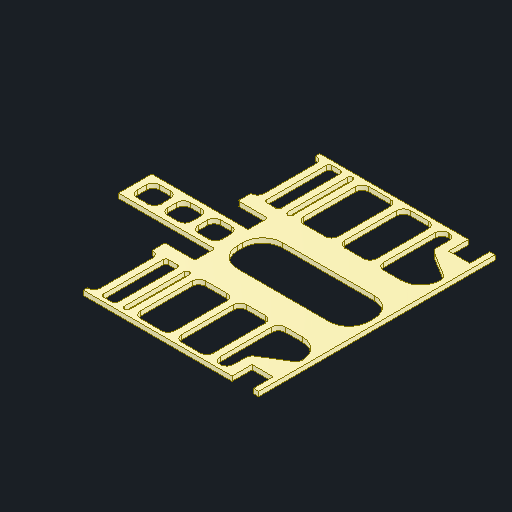
# Autodesk Inventor part: base
Saved by Autodesk Inventor 2023 (Build 270158000, 158)
## iProperties
Created: 2024-04-29
Part Number: base
Material: Nylon 6/6
Document SubType Name: Modeling
Designer: szymo
Density: 1.13 g/cm^3
Appearance: Nylon 6
Mass: 42.7646 g
Surface Area: 306.54 cm^2
Volume: 37.8447 cm^3
Author: szymo
Autodesk Inventor part; units mm, degrees
ref_plane "YZ Plane" through (0, 0, 0) normal (1, 0, 0) x (0, 1, 0)
ref_plane "XZ Plane" through (0, 0, 0) normal (0, 1, 0) x (-1, 0, 0)
ref_plane "XY Plane" through (0, 0, 0) normal (0, 0, 1) x (1, 0, 0)
sketch "Sketch1" plane through (0, 0, 0) normal (0, 1, 0) x (-1, 0, 0)
  line L0 (99, 89) -> (-99, 89)
  line L1 (-99, 89) -> (-99, -89)
  line L2 (-99, -89) -> (99, -89)
  line L3 (99, -89) -> (99, 89)
  line L4 (99, 89) -> (-99, -89) construction
  line L5 (-99, 89) -> (99, -89) construction
  line L6 (-99, 89) -> (-85, 89)
  line L7 (-85, 89) -> (-85, -89)
  line L8 (-85, -89) -> (-99, -89)
  line L9 (-99, -89) -> (-99, 89)
  line L10 (99, 89) -> (97, 89)
  line L11 (97, 89) -> (97, -89)
  line L12 (97, -89) -> (99, -89)
  line L13 (99, -89) -> (99, 89)
  line L14 (97, 33) -> (97, 35)
  line L15 (97, -33) -> (97, -35)
  line L16 (97, 32.8) -> (97, 35)
  line L17 (97, -32.8) -> (97, -35)
  line L18 (97, 89) -> (47, 89)
  line L19 (47, 89) -> (47, 30.5)
  line L20 (47, 30.5) -> (97, 30.5)
  line L21 (97, 30.5) -> (97, 89)
  line L22 (97, -89) -> (47, -89)
  line L23 (47, -89) -> (47, -30.5)
  line L24 (47, -30.5) -> (97, -30.5)
  line L25 (97, -30.5) -> (97, -89)
  line L26 (-81, 74) -> (-81, 89) projected
  line L27 (-81, 31) -> (-81, 55) projected
  line L28 (-81, -12) -> (-81, 12) projected
  line L29 (-81, -55) -> (-81, -31) projected
  line L30 (-81, -89) -> (-81, -74) projected
  arc A0 (-81, 74) -> (-79, 72) centre (-79, 74) ccw projected
  line L31 (-70, 72) -> (-79, 72) projected
  line L32 (-70, 57) -> (-70, 72) projected
  line L33 (-79, 57) -> (-70, 57) projected
  arc A1 (-79, 57) -> (-81, 55) centre (-79, 55) ccw projected
  arc A2 (-81, 31) -> (-79, 29) centre (-79, 31) ccw projected
  line L34 (-70, 29) -> (-79, 29) projected
  line L35 (-70, 14) -> (-70, 29) projected
  line L36 (-79, 14) -> (-70, 14) projected
  arc A3 (-79, 14) -> (-81, 12) centre (-79, 12) ccw projected
  arc A4 (-81, -12) -> (-79, -14) centre (-79, -12) ccw projected
  line L37 (-70, -14) -> (-79, -14) projected
  line L38 (-70, -29) -> (-70, -14) projected
  line L39 (-79, -29) -> (-70, -29) projected
  arc A5 (-79, -29) -> (-81, -31) centre (-79, -31) ccw projected
  arc A6 (-81, -55) -> (-79, -57) centre (-79, -55) ccw projected
  line L40 (-70, -57) -> (-79, -57) projected
  line L41 (-70, -72) -> (-70, -57) projected
  line L42 (-79, -72) -> (-70, -72) projected
  arc A7 (-79, -72) -> (-81, -74) centre (-79, -74) ccw projected
  circle A8 centre (-77, -64.5) radius 1.2295 projected
  circle A9 centre (-77, -21.5) radius 1.2295 projected
  circle A10 centre (-77, 21.5) radius 1.2295 projected
  circle A11 centre (-77, 64.5) radius 1.2295 projected
  line L43 (-65, 89) -> (-79, 89)
  line L44 (-79, 89) -> (-79, 75)
  line L45 (-79, 75) -> (-65, 75)
  line L46 (-65, 75) -> (-65, 89)
  line L47 (-65, 89) -> (-81, 89)
  line L48 (-81, 89) -> (-81, 74)
  line L49 (-81, 74) -> (-65, 74)
  line L50 (-65, 74) -> (-65, 89)
  line L51 (-99, 0) -> (97, 0)
  line L52 (0, 0) -> (-99, 0) construction
  line L53 (-65, -89) -> (-79, -89)
  line L54 (-79, -89) -> (-79, -75)
  line L55 (-79, -75) -> (-65, -75)
  line L56 (-65, -75) -> (-65, -89)
  line L57 (-65, -89) -> (-81, -89)
  line L58 (-81, -89) -> (-81, -74)
  line L59 (-81, -74) -> (-65, -74)
  line L60 (-65, -74) -> (-65, -89)
  line L61 (77.5, 29.5) -> (66.5, 29.5) projected
  line L62 (66.5, -29.5) -> (77.5, -29.5) projected
  point P0 (47, 89)
  point P1 (47, -89)
  point P2 (97, -30.5)
  point P3 (97, 30.5)
  point P4 (-81, -89)
  point P5 (-79, -74)
  dimension "d0" = 198
  dimension "d1" = 178
  dimension "d2" = 14
  dimension "d3" = 2
  dimension "d16" = 50
  dimension "d17" = 58.5
  dimension "d18" = 50
  dimension "d19" = 58.5
  dimension "d22" = 14
  dimension "d23" = 14
  dimension "d24" = 2
  dimension "d25" = 1
  dimension "d26" = 2
  dimension "d87" = 1
  dimension "d88" = 1
  constraints: 88 end point, 14 parallel, 10 symmetric about line, 8 perpendicular, 8 point on line, 7 horizontal, 4 midpoint, 2 collinear
  measures "d0" distance of L2.end L1.end
  measures "d1" distance of L1.end L0.end
  measures "d2" distance of L7.end L8.end
  measures "d3" distance of L12.end L11.end
  measures "d16" distance of L20.end L19.end
  measures "d17" distance of L19.end L18.end
  measures "d18" distance of L23.end L24.end
  measures "d19" distance of L22.end L23.end
  measures "d22" distance of L45.end L44.end
  measures "d23" distance of L44.end L43.end
  measures "d24" distance between parallel lines of L26 L44
  measures "d25" distance between parallel lines of L45 L49
  measures "d26" distance between parallel lines of L31 L49
  measures "d87" distance between parallel lines of L20 L61
  measures "d88" distance between parallel lines of L24 L62
extrude "Extrusion1" add sketch "Sketch1" along normal blind 3.5 contours L19 L20 L11 L51 L28 A3 L36 L35 L34 A2 L27 A1 L33 L32 L31 A0 L49 L50 L46 L0 | L2 L56 L60 L59 A7 L42 L41 L40 A6 L29 A5 L39 L38 L37 A4 L28 L51 L11 L24 L23 | L26 A0 L31 L32 L33 A1 L27 A2 L34 L35 L36 A3 L28 L51 L7 L0 | L28 A4 L37 L38 L39 A5 L29 A6 L40 L41 L42 A7 L30 L2 L7 L51 | A8 | A9 | A10 | A11
sketch "Sketch16" plane through (0, 0, 0) normal (0, 1, 0) x (1, 0, 0)
  line L0 (-36.8852, -42) -> (-31.5, -42) construction
  line L1 (-31.5, -42) -> (-26.1148, -42) construction
  line L2 (-26.1148, -42) -> (-26.1148, -69.7) construction
  line L3 (-26.1148, -69.7) -> (-36.8852, -69.7) construction
  line L4 (-36.8852, -69.7) -> (-36.8852, -42) construction
  line L5 (-26.1148, 42) -> (-31.5, 42) construction
  line L6 (-31.5, 42) -> (-36.8852, 42) construction
  line L7 (-36.8852, 42) -> (-36.8852, 69.7) construction
  line L8 (-36.8852, 69.7) -> (-26.1148, 69.7) construction
  line L9 (-26.1148, 69.7) -> (-26.1148, 42) construction
  line L10 (-24.5, 21) -> (-24.5, 27.5) construction
  line L11 (-24.5, 27.5) -> (-36.7968, 27.5) construction
  spline S0 degree 3 poles (-38.9709, 26) (-38.9452, 26.0786) (-38.9168, 26.1547) (-38.7761, 26.4593) (-38.5883, 26.7067) (-38.1939, 27.0666) (-37.9122, 27.2391) (-37.3982, 27.4381) (-37.0728, 27.5) (-36.7968, 27.5) knots 0 0 0 0 0.086487 0.086487 0.378353 0.378353 0.688736 0.688736 1 1 1 1 construction
  line L12 (-38.9709, 26) -> (-45.6477, 26) construction
  spline S1 degree 3 poles (-45.6477, 26) (-45.6733, 26.0786) (-45.7018, 26.1547) (-45.8425, 26.4593) (-46.0302, 26.7067) (-46.4247, 27.0666) (-46.7063, 27.2391) (-47.2204, 27.4381) (-47.5457, 27.5) (-47.8217, 27.5) knots 0 0 0 0 0.086487 0.086487 0.378353 0.378353 0.688736 0.688736 1 1 1 1 construction
  line L13 (-47.8217, 27.5) -> (-65.1591, 27.5) construction
  spline S2 degree 3 poles (-68.2583, 26) (-68.2382, 26.0379) (-68.2174, 26.0746) (-68.0344, 26.3642) (-67.7636, 26.6069) (-67.1915, 26.9981) (-66.7665, 27.1943) (-66.018, 27.4248) (-65.5523, 27.5) (-65.1591, 27.5) knots 0 0 0 0 0.035027 0.035027 0.30423 0.30423 0.650773 0.650773 1 1 1 1 construction
  line L14 (-68.2583, 26) -> (-75.7417, 26) construction
  spline S3 degree 3 poles (-75.7417, 26) (-75.7753, 26.0631) (-75.8128, 26.1246) (-76.0566, 26.4695) (-76.3938, 26.7337) (-77.0078, 27.0936) (-77.4015, 27.2556) (-78.0794, 27.4407) (-78.4928, 27.5) (-78.8409, 27.5) knots 0 0 0 0 0.058061 0.058061 0.375369 0.375369 0.690666 0.690666 1 1 1 1 construction
  line L15 (-78.8409, 27.5) -> (-92, 27.5) construction
  arc A0 (-92, 27.5) -> (-92.866, 27) centre (-92, 26.5) ccw construction
  arc A1 (-93.7321, 26.5) -> (-92.866, 27) centre (-93.7321, 27.5) ccw construction
  line L16 (-93.7321, 26.5) -> (-97, 26.5) construction
  line L17 (-97, 30.5) -> (-97, 26.5) construction
  line L18 (-97, 30.5) -> (-18, 30.5) construction
  line L19 (-18, 30.5) -> (-18, 21) construction
  line L20 (-18, 21) -> (-24.5, 21) construction
  circle A2 centre (-21.25, 24.25) radius 1.8 construction
  circle A3 centre (-94, 10.5) radius 1.4 construction
  circle A4 centre (-21.25, 15.75) radius 1.8 construction
  line L21 (-37.4639, 12.5) -> (-24.5, 12.5) construction
  line L22 (-24.5, 12.5) -> (-24.5, 19) construction
  line L23 (-24.5, 19) -> (-18, 19) construction
  line L24 (-18, 8.5) -> (-18, 19) construction
  line L25 (-97, 8.5) -> (-18, 8.5) construction
  line L26 (-97, 8.5) -> (-97, 12.5) construction
  line L27 (-97, 12.5) -> (-76.3529, 12.5) construction
  line L28 (-76.3529, 12.5) -> (-73.0371, 12.5) construction
  line L29 (-73.0371, 12.5) -> (-72, 12.5) construction
  line L30 (-72, 12.5) -> (-70.9629, 12.5) construction
  line L31 (-70.9629, 12.5) -> (-67.6471, 12.5) construction
  line L32 (-67.6471, 12.5) -> (-47.1547, 12.5) construction
  spline S4 degree 3 poles (-45.6477, 13) (-45.8385, 12.8633) (-46.0608, 12.7418) (-46.5335, 12.5634) (-46.8696, 12.5) (-47.1547, 12.5) knots 0 0 0 0 0.435873 0.435873 1 1 1 1 construction
  line L33 (-43.2606, 13) -> (-45.6477, 13) construction
  spline S5 degree 3 poles (-43.2606, 13) (-43.1675, 13) (-43.0559, 12.9938) (-42.7588, 12.9716) (-42.5141, 12.9484) (-42.1044, 12.9484) (-41.8597, 12.9716) (-41.5626, 12.9938) (-41.4511, 13) (-41.358, 13) knots 0 0 0 0 0.156235 0.156235 0.5 0.5 0.843765 0.843765 1 1 1 1 construction
  line L34 (-38.9709, 13) -> (-41.358, 13) construction
  spline S6 degree 3 poles (-38.9709, 13) (-38.7801, 12.8633) (-38.5578, 12.7418) (-38.085, 12.5634) (-37.7489, 12.5) (-37.4639, 12.5) knots 0 0 0 0 0.435873 0.435873 1 1 1 1 construction
  circle A5 centre (-94, -10.5) radius 1.4 construction
  circle A6 centre (-21.25, -15.75) radius 1.8 construction
  line L35 (-37.4639, -12.5) -> (-24.5, -12.5) construction
  spline S7 degree 3 poles (-38.9709, -13) (-38.7801, -12.8633) (-38.5578, -12.7418) (-38.085, -12.5634) (-37.7489, -12.5) (-37.4639, -12.5) knots 0 0 0 0 0.435873 0.435873 1 1 1 1 construction
  line L36 (-38.9709, -13) -> (-41.358, -13) construction
  spline S8 degree 3 poles (-43.2606, -13) (-43.1675, -13) (-43.0559, -12.9938) (-42.7588, -12.9716) (-42.5141, -12.9484) (-42.1044, -12.9484) (-41.8597, -12.9716) (-41.5626, -12.9938) (-41.4511, -13) (-41.358, -13) knots 0 0 0 0 0.156235 0.156235 0.5 0.5 0.843765 0.843765 1 1 1 1 construction
  line L37 (-43.2606, -13) -> (-45.6477, -13) construction
  spline S9 degree 3 poles (-45.6477, -13) (-45.8385, -12.8633) (-46.0608, -12.7418) (-46.5335, -12.5634) (-46.8696, -12.5) (-47.1547, -12.5) knots 0 0 0 0 0.435873 0.435873 1 1 1 1 construction
  line L38 (-67.6471, -12.5) -> (-47.1547, -12.5) construction
  line L39 (-70.9629, -12.5) -> (-67.6471, -12.5) construction
  line L40 (-72, -12.5) -> (-70.9629, -12.5) construction
  line L41 (-73.0371, -12.5) -> (-72, -12.5) construction
  line L42 (-76.3529, -12.5) -> (-73.0371, -12.5) construction
  line L43 (-97, -12.5) -> (-76.3529, -12.5) construction
  line L44 (-97, -8.5) -> (-97, -12.5) construction
  line L45 (-97, -8.5) -> (-18, -8.5) construction
  line L46 (-18, -8.5) -> (-18, -19) construction
  line L47 (-24.5, -19) -> (-18, -19) construction
  line L48 (-24.5, -12.5) -> (-24.5, -19) construction
  line L49 (-24.5, -21) -> (-24.5, -27.5) construction
  line L50 (-18, -21) -> (-24.5, -21) construction
  line L51 (-18, -30.5) -> (-18, -21) construction
  line L52 (-97, -30.5) -> (-18, -30.5) construction
  line L53 (-97, -30.5) -> (-97, -26.5) construction
  line L54 (-93.7321, -26.5) -> (-97, -26.5) construction
  arc A7 (-92.866, -27) -> (-93.7321, -26.5) centre (-93.7321, -27.5) ccw construction
  arc A8 (-92.866, -27) -> (-92, -27.5) centre (-92, -26.5) ccw construction
  line L55 (-78.8409, -27.5) -> (-92, -27.5) construction
  spline S10 degree 3 poles (-75.7417, -26) (-75.7753, -26.0631) (-75.8128, -26.1246) (-76.0566, -26.4695) (-76.3938, -26.7337) (-77.0078, -27.0936) (-77.4015, -27.2556) (-78.0794, -27.4407) (-78.4928, -27.5) (-78.8409, -27.5) knots 0 0 0 0 0.058061 0.058061 0.375369 0.375369 0.690666 0.690666 1 1 1 1 construction
  line L56 (-68.2583, -26) -> (-75.7417, -26) construction
  spline S11 degree 3 poles (-68.2583, -26) (-68.2382, -26.0379) (-68.2174, -26.0746) (-68.0344, -26.3642) (-67.7636, -26.6069) (-67.1915, -26.9981) (-66.7665, -27.1943) (-66.018, -27.4248) (-65.5523, -27.5) (-65.1591, -27.5) knots 0 0 0 0 0.035027 0.035027 0.30423 0.30423 0.650773 0.650773 1 1 1 1 construction
  line L57 (-47.8217, -27.5) -> (-65.1591, -27.5) construction
  spline S12 degree 3 poles (-45.6477, -26) (-45.6733, -26.0786) (-45.7018, -26.1547) (-45.8425, -26.4593) (-46.0302, -26.7067) (-46.4247, -27.0666) (-46.7063, -27.2391) (-47.2204, -27.4381) (-47.5457, -27.5) (-47.8217, -27.5) knots 0 0 0 0 0.086487 0.086487 0.378353 0.378353 0.688736 0.688736 1 1 1 1 construction
  line L58 (-38.9709, -26) -> (-45.6477, -26) construction
  spline S13 degree 3 poles (-38.9709, -26) (-38.9452, -26.0786) (-38.9168, -26.1547) (-38.7761, -26.4593) (-38.5883, -26.7067) (-38.1939, -27.0666) (-37.9122, -27.2391) (-37.3982, -27.4381) (-37.0728, -27.5) (-36.7968, -27.5) knots 0 0 0 0 0.086487 0.086487 0.378353 0.378353 0.688736 0.688736 1 1 1 1 construction
  line L59 (-24.5, -27.5) -> (-36.7968, -27.5) construction
  circle A9 centre (-21.25, -24.25) radius 1.8 construction
  line L60 (14.0482, -86) -> (-12.0482, -86) construction
  arc A10 (14, -85.6932) -> (14.0482, -86) centre (15, -85.6932) ccw construction
  line L61 (14, -82) -> (14, -85.6932) construction
  arc A11 (15, -81) -> (14, -82) centre (15, -82) ccw construction
  line L62 (18, -81) -> (15, -81) construction
  arc A12 (19, -82) -> (18, -81) centre (18, -82) ccw construction
  line L63 (19, -85.6932) -> (19, -82) construction
  arc A13 (18.9518, -86) -> (19, -85.6932) centre (18, -85.6932) ccw construction
  line L64 (42.9867, -86) -> (18.9518, -86) construction
  arc A14 (42.9385, -85.6932) -> (42.9867, -86) centre (43.9385, -85.6932) ccw construction
  line L65 (42.9385, -82) -> (42.9385, -85.6932) construction
  arc A15 (43.9385, -81) -> (42.9385, -82) centre (43.9385, -82) ccw construction
  line L66 (46.9385, -81) -> (43.9385, -81) construction
  arc A16 (47.9385, -82) -> (46.9385, -81) centre (46.9385, -82) ccw construction
  line L67 (47.9385, -85.6932) -> (47.9385, -82) construction
  arc A17 (47.8903, -86) -> (47.9385, -85.6932) centre (46.9385, -85.6932) ccw construction
  line L68 (58, -86) -> (47.8903, -86) construction
  line L69 (58, -74) -> (58, -86) construction
  line L70 (58, -69) -> (58, -74) construction
  line L71 (65, -69) -> (58, -69) construction
  line L72 (65, -71.75) -> (65, -69) construction
  arc A18 (65, -71.75) -> (68.2269, -75.875) centre (69.25, -71.75) ccw construction
  line L73 (68.2269, -76) -> (68.2269, -75.875) construction
  line L74 (70.25, -76) -> (68.2269, -76) construction
  arc A19 (74.5, -80.25) -> (70.25, -76) centre (70.25, -80.25) ccw construction
  line L75 (74.5, -83.75) -> (74.5, -80.25) construction
  arc A20 (74.5, -83.75) -> (78.75, -88) centre (78.75, -83.75) ccw construction
  line L76 (80, -88) -> (78.75, -88) construction
  line L77 (80, -89) -> (80, -88) construction
  line L78 (-47, -89) -> (80, -89) construction
  line L79 (-47, -89) -> (-47, -86) construction
  line L80 (-41.1603, -86) -> (-47, -86) construction
  arc A21 (-41.1603, -86) -> (-40.1603, -85) centre (-41.1603, -85) ccw construction
  line L81 (-40.1603, -85) -> (-40.1603, -81.6) construction
  line L82 (-31.5, -81.6) -> (-40.1603, -81.6) construction
  line L83 (-31.5, -88) -> (-31.5, -81.6) construction
  line L84 (-22.8397, -81.6) -> (-31.5, -81.6) construction
  line L85 (-22.8397, -85) -> (-22.8397, -81.6) construction
  arc A22 (-22.8397, -85) -> (-21.8397, -86) centre (-21.8397, -85) ccw construction
  line L86 (-17, -86) -> (-21.8397, -86) construction
  line L87 (-17, -80.9087) -> (-17, -86) construction
  arc A23 (-16, -79.9087) -> (-17, -80.9087) centre (-16, -80.9087) ccw construction
  line L88 (-13, -79.9087) -> (-16, -79.9087) construction
  arc A24 (-12, -80.9087) -> (-13, -79.9087) centre (-13, -80.9087) ccw construction
  line L89 (-12, -85.6932) -> (-12, -80.9087) construction
  arc A25 (-12.0482, -86) -> (-12, -85.6932) centre (-13, -85.6932) ccw construction
  circle A26 centre (16.5, -83.5) radius 1.15 construction
  circle A27 centre (-14.5, -82.4087) radius 1.15 construction
  circle A28 centre (45.4385, -83.5) radius 1.15 construction
  circle A29 centre (70, -80) radius 1.75 construction
  circle A30 centre (61.5, -84.5) radius 1.8 construction
  circle A31 centre (18.4119, -29.75) radius 1.55 construction
  circle A32 centre (43.009, -29.75) radius 1.55 construction
  circle A33 centre (17.4, -24.1) radius 1.6 construction
  circle A34 centre (65.6, -24.1) radius 1.6 construction
  circle A35 centre (-12.1414, -28.5) radius 1.8 construction
  circle A36 centre (76.75, -33.75) radius 1.8 construction
  arc A37 (69.6, -27.9275) -> (73.5136, -30.785) centre (72.6, -27.9275) ccw construction
  arc A38 (75.3408, -30.5) -> (73.5136, -30.785) centre (75.3408, -36.5) ccw construction
  line L90 (80, -30.5) -> (75.3408, -30.5) construction
  line L91 (80, -37) -> (80, -30.5) construction
  line L92 (52.4519, -37) -> (80, -37) construction
  line L93 (52.4519, -36) -> (52.4519, -37) construction
  line L94 (-47, -37) -> (52.4519, -37) construction
  line L95 (-47, -37) -> (-47, -32) construction
  line L96 (-20.5, -32) -> (-47, -32) construction
  arc A39 (-20.5, -32) -> (-16.5, -28) centre (-20.5, -28) ccw construction
  line L97 (-16.5, -28) -> (-16.5, -25) construction
  line L98 (-7.7828, -25) -> (-16.5, -25) construction
  arc A40 (-7.7828, -25) -> (-0.7828, -32) centre (-0.7828, -25) ccw construction
  line L99 (8.2992, -32) -> (-0.7828, -32) construction
  arc A41 (8.2992, -32) -> (14.0533, -27.7) centre (8.2992, -26) ccw construction
  line L100 (14.0533, -20.1) -> (14.0533, -27.7) construction
  line L101 (22.7705, -20.1) -> (14.0533, -20.1) construction
  line L102 (22.7705, -27.7) -> (22.7705, -20.1) construction
  arc A42 (22.7705, -27.7) -> (28.5247, -32) centre (28.5247, -26) ccw construction
  line L103 (32.8963, -32) -> (28.5247, -32) construction
  arc A43 (32.8963, -32) -> (38.6504, -27.7) centre (32.8963, -26) ccw construction
  line L104 (47.3676, -27.7) -> (38.6504, -27.7) construction
  arc A44 (47.3676, -27.7) -> (53.1217, -32) centre (53.1217, -26) ccw construction
  line L105 (56.6, -32) -> (53.1217, -32) construction
  arc A45 (56.6, -32) -> (61.6, -27) centre (56.6, -27) ccw construction
  line L106 (61.6, -20.1) -> (61.6, -27) construction
  line L107 (69.6, -20.1) -> (61.6, -20.1) construction
  line L108 (69.6, -27.9275) -> (69.6, -20.1) construction
  circle A46 centre (70, 83) radius 1.75 construction
  line L109 (14.0482, 86) -> (-12.0482, 86) construction
  arc A47 (-12, 85.6932) -> (-12.0482, 86) centre (-13, 85.6932) ccw construction
  line L110 (-12, 85.6932) -> (-12, 80.9087) construction
  arc A48 (-13, 79.9087) -> (-12, 80.9087) centre (-13, 80.9087) ccw construction
  line L111 (-13, 79.9087) -> (-16, 79.9087) construction
  arc A49 (-17, 80.9087) -> (-16, 79.9087) centre (-16, 80.9087) ccw construction
  line L112 (-17, 80.9087) -> (-17, 86) construction
  line L113 (-17, 86) -> (-21.8397, 86) construction
  arc A50 (-21.8397, 86) -> (-22.8397, 85) centre (-21.8397, 85) ccw construction
  line L114 (-22.8397, 85) -> (-22.8397, 81.6) construction
  line L115 (-22.8397, 81.6) -> (-31.5, 81.6) construction
  line L116 (-31.5, 88) -> (-31.5, 81.6) construction
  line L117 (-31.5, 81.6) -> (-40.1603, 81.6) construction
  line L118 (-40.1603, 85) -> (-40.1603, 81.6) construction
  arc A51 (-40.1603, 85) -> (-41.1603, 86) centre (-41.1603, 85) ccw construction
  line L119 (-41.1603, 86) -> (-47, 86) construction
  line L120 (-47, 89) -> (-47, 86) construction
  line L121 (-47, 89) -> (80, 89) construction
  line L122 (80, 89) -> (80, 88) construction
  line L123 (80, 88) -> (78.75, 88) construction
  arc A52 (78.75, 88) -> (74.5, 83.75) centre (78.75, 83.75) ccw construction
  line L124 (74.5, 83.75) -> (74.5, 80.25) construction
  arc A53 (70.25, 76) -> (74.5, 80.25) centre (70.25, 80.25) ccw construction
  line L125 (70.25, 76) -> (68.6269, 76) construction
  line L126 (68.6269, 76) -> (68.6269, 75.875) construction
  arc A54 (68.6269, 75.875) -> (65.4, 71.75) centre (69.65, 71.75) ccw construction
  line L127 (65.4, 71.75) -> (65.4, 69) construction
  line L128 (65.4, 69) -> (58.4, 69) construction
  line L129 (58.4, 69) -> (58.4, 74) construction
  line L130 (58.4, 74) -> (58.4, 86) construction
  line L131 (58.4, 86) -> (47.8903, 86) construction
  arc A55 (47.9385, 85.6932) -> (47.8903, 86) centre (46.9385, 85.6932) ccw construction
  line L132 (47.9385, 85.6932) -> (47.9385, 82) construction
  arc A56 (46.9385, 81) -> (47.9385, 82) centre (46.9385, 82) ccw construction
  line L133 (46.9385, 81) -> (43.9385, 81) construction
  arc A57 (42.9385, 82) -> (43.9385, 81) centre (43.9385, 82) ccw construction
  line L134 (42.9385, 82) -> (42.9385, 85.6932) construction
  arc A58 (42.9867, 86) -> (42.9385, 85.6932) centre (43.9385, 85.6932) ccw construction
  line L135 (42.9867, 86) -> (18.9518, 86) construction
  arc A59 (19, 85.6932) -> (18.9518, 86) centre (18, 85.6932) ccw construction
  line L136 (19, 85.6932) -> (19, 82) construction
  arc A60 (18, 81) -> (19, 82) centre (18, 82) ccw construction
  line L137 (18, 81) -> (15, 81) construction
  arc A61 (14, 82) -> (15, 81) centre (15, 82) ccw construction
  line L138 (14, 82) -> (14, 85.6932) construction
  arc A62 (14.0482, 86) -> (14, 85.6932) centre (15, 85.6932) ccw construction
  circle A63 centre (16.5, 83.5) radius 1.15 construction
  circle A64 centre (-14.5, 82.4087) radius 1.15 construction
  circle A65 centre (45.4385, 83.5) radius 1.15 construction
  circle A66 centre (61.9, 84.5) radius 1.8 construction
  circle A67 centre (18.4119, 29.75) radius 1.55 construction
  circle A68 centre (43.009, 29.75) radius 1.55 construction
  circle A69 centre (17.4, 24.1) radius 1.6 construction
  circle A70 centre (65.6, 24.1) radius 1.6 construction
  circle A71 centre (-12.1414, 28.5) radius 1.8 construction
  circle A72 centre (76.75, 33.75) radius 1.8 construction
  arc A73 (73.5136, 30.785) -> (69.6, 27.9275) centre (72.6, 27.9275) ccw construction
  line L139 (69.6, 27.9275) -> (69.6, 20.1) construction
  line L140 (69.6, 20.1) -> (61.6, 20.1) construction
  line L141 (61.6, 20.1) -> (61.6, 27) construction
  arc A74 (61.6, 27) -> (56.6, 32) centre (56.6, 27) ccw construction
  line L142 (56.6, 32) -> (53.1217, 32) construction
  arc A75 (53.1217, 32) -> (47.3676, 27.7) centre (53.1217, 26) ccw construction
  line L143 (47.3676, 27.7) -> (38.6504, 27.7) construction
  arc A76 (38.6504, 27.7) -> (32.8963, 32) centre (32.8963, 26) ccw construction
  line L144 (32.8963, 32) -> (28.5247, 32) construction
  arc A77 (28.5247, 32) -> (22.7705, 27.7) centre (28.5247, 26) ccw construction
  line L145 (22.7705, 27.7) -> (22.7705, 20.1) construction
  line L146 (22.7705, 20.1) -> (14.0533, 20.1) construction
  line L147 (14.0533, 20.1) -> (14.0533, 27.7) construction
  arc A78 (14.0533, 27.7) -> (8.2992, 32) centre (8.2992, 26) ccw construction
  line L148 (8.2992, 32) -> (-0.7828, 32) construction
  arc A79 (-0.7828, 32) -> (-7.7828, 25) centre (-0.7828, 25) ccw construction
  line L149 (-7.7828, 25) -> (-16.5, 25) construction
  line L150 (-16.5, 28) -> (-16.5, 25) construction
  arc A80 (-16.5, 28) -> (-20.5, 32) centre (-20.5, 28) ccw construction
  line L151 (-20.5, 32) -> (-47, 32) construction
  line L152 (-47, 37) -> (-47, 32) construction
  line L153 (-47, 37) -> (52.4519, 37) construction
  line L154 (52.4519, 36) -> (52.4519, 37) construction
  line L155 (52.4519, 37) -> (80, 37) construction
  line L156 (80, 37) -> (80, 30.5) construction
  line L157 (80, 30.5) -> (75.3408, 30.5) construction
  arc A81 (73.5136, 30.785) -> (75.3408, 30.5) centre (75.3408, 36.5) ccw construction
  line L158 (-15.5, 70.1149) -> (50.5, 70.1149) construction
  line L159 (50.5, 70.1149) -> (50.5, 40.1149) construction
  line L160 (-15.5, 40.1149) -> (50.5, 40.1149) construction
  line L161 (-15.5, 70.1149) -> (-15.5, 40.1149) construction
  line L162 (50.5, -71.1831) -> (-15.5, -71.1831) construction
  line L163 (-15.5, -71.1831) -> (-15.5, -41.1831) construction
  line L164 (50.5, -41.1831) -> (-15.5, -41.1831) construction
  line L165 (50.5, -71.1831) -> (50.5, -41.1831) construction
  line L166 (85, 89) -> (99, 89) construction
  line L167 (99, 89) -> (99, -89) construction
  line L168 (85, -89) -> (99, -89) construction
  line L169 (85, 89) -> (85, -89) construction
  circle A82 centre (77, -21.5) radius 1.2295 construction
  circle A83 centre (77, 64.5) radius 1.2295 construction
  circle A84 centre (77, 21.5) radius 1.2295 construction
  circle A85 centre (77, -64.5) radius 1.2295 construction
  line L170 (70, 72) -> (79, 72)
  arc A86 (79, 72) -> (81, 74) centre (79, 74) ccw
  line L171 (81, 74) -> (81, 89) construction
  line L172 (81, 89) -> (85, 89)
  line L173 (85, 89) -> (85, -89)
  line L174 (81, -89) -> (85, -89)
  line L175 (81, -89) -> (81, -74) construction
  arc A87 (81, -74) -> (79, -72) centre (79, -74) ccw
  line L176 (79, -72) -> (70, -72)
  line L177 (70, -57) -> (70, -72)
  line L178 (70, -57) -> (79, -57)
  arc A88 (79, -57) -> (81, -55) centre (79, -55) ccw
  line L179 (81, -55) -> (81, -31)
  arc A89 (81, -31) -> (79, -29) centre (79, -31) ccw
  line L180 (79, -29) -> (70, -29)
  line L181 (70, -14) -> (70, -29)
  line L182 (70, -14) -> (79, -14)
  arc A90 (79, -14) -> (81, -12) centre (79, -12) ccw
  line L183 (81, -12) -> (81, 12)
  arc A91 (81, 12) -> (79, 14) centre (79, 12) ccw
  line L184 (79, 14) -> (70, 14)
  line L185 (70, 29) -> (70, 14)
  line L186 (70, 29) -> (79, 29)
  arc A92 (79, 29) -> (81, 31) centre (79, 31) ccw
  line L187 (81, 31) -> (81, 55)
  arc A93 (81, 55) -> (79, 57) centre (79, 55) ccw
  line L188 (79, 57) -> (70, 57)
  line L189 (70, 72) -> (70, 57)
  line L190 (81, 74) -> (65, 74)
  line L191 (65, 74) -> (65, 89)
  line L192 (65, -89) -> (65, -74)
  line L193 (65, -74) -> (81, -74)
  line L194 (81, -74) -> (81, -89)
  line L195 (81, 89) -> (81, 74)
  line L196 (65, 89) -> (-47, 89)
  line L197 (-47, 86) -> (-47, 89)
  line L198 (-47, 86) -> (58.4, 86)
  line L199 (58.4, 86) -> (58.4, 69)
  line L200 (58.4, 69) -> (81, 55)
  line L201 (65, -89) -> (-47, -89)
  line L202 (-47, -86) -> (-47, -89)
  line L203 (58, -86) -> (-47, -86)
  line L204 (58, -86) -> (58, -69)
  line L205 (58, -69) -> (81, -55)
  line L206 (81, 37) -> (-47, 37)
  line L207 (81, -37) -> (-47, -37)
  line L208 (-47, -37) -> (-47, -27.5)
  line L209 (-47, -27.5) -> (-24.5, -27.5)
  line L210 (-47, 37) -> (-47, 27.5)
  line L211 (-47, 27.5) -> (-24.5, 27.5)
  line L212 (-24.5, 27.5) -> (-24.5, 12.5)
  line L213 (-24.5, 12.5) -> (-97, 12.5)
  line L214 (-97, 12.5) -> (-97, -12.5)
  line L215 (-97, -12.5) -> (-24.5, -12.5)
  line L216 (-24.5, -12.5) -> (-24.5, -27.5)
  line L217 (-92, 8.5) -> (-74, 8.5)
  line L218 (-74, 8.5) -> (-74, -8.5)
  line L219 (-74, -8.5) -> (-92, -8.5)
  line L220 (-92, -8.5) -> (-92, 8.5)
  line L221 (-69, 8.5) -> (-51, 8.5)
  line L222 (-51, 8.5) -> (-51, -8.5)
  line L223 (-51, -8.5) -> (-69, -8.5)
  line L224 (-69, -8.5) -> (-69, 8.5)
  line L225 (-46, 8.5) -> (-28, 8.5)
  line L226 (-28, 8.5) -> (-28, -8.5)
  line L227 (-28, -8.5) -> (-46, -8.5)
  line L228 (-46, -8.5) -> (-46, 8.5)
  line L229 (70, 17) -> (-18, 17)
  line L230 (70, -17) -> (-18, -17)
  line L231 (-36.8852, 37) -> (-41.8852, 37)
  line L232 (-41.8852, 37) -> (-41.8852, 86)
  line L233 (-41.8852, 86) -> (-36.8852, 86)
  line L234 (-36.8852, 86) -> (-36.8852, 37)
  line L235 (-21.1148, 37) -> (-26.1148, 37)
  line L236 (-26.1148, 37) -> (-26.1148, 86)
  line L237 (-26.1148, 86) -> (-21.1148, 86)
  line L238 (-21.1148, 86) -> (-21.1148, 37)
  line L239 (-97, 30.5) -> (-97, -30.5)
  line L240 (-47, 30.5) -> (-97, 30.5)
  line L241 (-97, -30.5) -> (-47, -30.5)
  line L242 (-47, -30.5) -> (-47, -89)
  line L243 (-47, 89) -> (-47, 30.5)
  line L244 (-18, 17) -> (-18, -17)
  line L245 (-18, 10) -> (-11, 17)
  line L246 (-18, -10) -> (-11, -17)
  line L247 (81, 10) -> (74, 17)
  line L248 (81, -10) -> (74, -17)
  line L249 (74, 37) -> (81, 44)
  line L250 (74, -37) -> (81, -44)
  line L251 (-17, 86) -> (-17, 37)
  line L252 (-12, 86) -> (-12, 37)
  line L253 (14.0482, 86) -> (14.0482, 37)
  line L254 (19, 86) -> (19, 37)
  line L255 (42.9385, 86) -> (42.9385, 37)
  line L256 (47.9385, 86) -> (47.9385, 37)
  line L257 (-41.8852, -37) -> (-36.8852, -37)
  line L258 (-36.8852, -37) -> (-36.8852, -86)
  line L259 (-36.8852, -86) -> (-41.8852, -86)
  line L260 (-41.8852, -86) -> (-41.8852, -37)
  line L261 (-26.1148, -37) -> (-21.1148, -37)
  line L262 (-21.1148, -37) -> (-21.1148, -86)
  line L263 (-21.1148, -86) -> (-26.1148, -86)
  line L264 (-26.1148, -86) -> (-26.1148, -37)
  line L265 (-17, -86) -> (-17, -37)
  line L266 (-12, -86) -> (-12, -37)
  line L267 (14, -86) -> (14, -37)
  line L268 (19, -86) -> (19, -37)
  line L269 (42.9385, -86) -> (42.9385, -37)
  line L270 (47.9385, -86) -> (47.9385, -37)
  line L271 (74, 17) -> (70, 17)
  line L272 (74, -17) -> (70, -17)
  point P0 (0, 0)
  point P1 (70, -61.6957)
  point P2 (77.7143, -57)
  point P3 (77.7714, 57)
  point P4 (70, 61.8142)
  point P5 (70, -16)
  point P6 (77, -14)
  point P7 (77, 14)
  point P8 (70, 16)
  dimension "d202" = 5
  dimension "d204" = 5
  dimension "d205" = 5
  dimension "d206" = 18
  dimension "d207" = 18
  dimension "d208" = 18
  dimension "d209" = 20
  dimension "d210" = 20
  dimension "d211" = 5
  dimension "d212" = 5
  dimension "d215" = 45
  dimension "d216" = 45
  dimension "d217" = 7
  dimension "d218" = 7
  dimension "d219" = 10
  dimension "d220" = 45
  dimension "d221" = 45
  dimension "d222" = 7
  dimension "d223" = 7
  dimension "d224" = 45
  dimension "d225" = 45
  dimension "d226" = 7
  dimension "d227" = 7
  dimension "d228" = 5
  dimension "d229" = 4.9518
  dimension "d230" = 5
  dimension "d231" = 5
  dimension "d232" = 5
  dimension "d233" = 5
  dimension "d234" = 5
  dimension "d235" = 5
  constraints: 159 end point, 39 point on line, 19 horizontal, 17 perpendicular, 15 collinear, 15 parallel, 10 vertical, 44 other
  measures "d202" distance between parallel lines of L214 L220
  measures "d204" distance between parallel lines of L222 L228
  measures "d205" distance between parallel lines of L218 L224
  measures "d206" distance between parallel lines of L220 L218
  measures "d207" distance between parallel lines of L224 L222
  measures "d208" distance between parallel lines of L228 L226
  measures "d209" distance between parallel lines of L153 L229
  measures "d210" distance between parallel lines of L94 L230
  measures "d211" distance of L232.end L233.end
  measures "d212" distance between parallel lines of L236 L238
  measures "d215" angle of L245 L244
  measures "d216" angle of L244 L246
  measures "d217" distance of L229.end L245.start
  measures "d218" distance of L246.start L230.end
  measures "d219" distance between parallel lines of L226 L244
  measures "d220" angle of L229 L247
  measures "d221" angle of L248 L230
  measures "d222" distance from line of L230 L248.start
  measures "d223" distance from line of L247.start L229
  measures "d224" angle to the sketch x axis of L249
  measures "d225" angle of L92 L250
  measures "d228" distance between parallel lines of L255 L256
  measures "d229" distance between parallel lines of L253 L254
  measures "d230" distance between parallel lines of L251 L252
  measures "d231" distance between parallel lines of L264 L262
  measures "d232" distance between parallel lines of L260 L258
  measures "d233" distance between parallel lines of L265 L266
  measures "d234" distance between parallel lines of L267 L268
  measures "d235" distance between parallel lines of L269 L270
extrude "zeberka" cut sketch "Sketch16" along normal up to next contours L200 L188 L189 | L189 L188 L200 L187 L249 L206 L256 L198 L199 | L255 L206 L254 L198 | L198 L232 L206 L243 | L253 L206 L252 L198 | L198 L236 L206 L234 | L210 L211 L212 L213 L239 L240 | L251 L206 L238 L198 | L271 L247 L184 L185 | L185 L184 L247 L183 L248 L182 L181 L230 L246 L244 L245 L229 | L205 L204 L203 L270 L207 L250 L179 L178 L177 | L177 L178 L205 | L215 L216 L209 L208 L241 L239 | L242 L207 L260 L203 | L258 L207 L264 L203 | L203 L268 L207 L269 | L248 L272 L181 L182 | L262 L207 L265 L203 | L203 L266 L207 L267 | L217 L218 L219 L220 | L221 L222 L223 L224 | L225 L226 L227 L228
fillet "Fillet14" radius 5 12 edges at (-92, 1.75, -8.5) (-92, 1.75, 8.5) (-74, 1.75, 8.5) (-74, 1.75, -8.5) (-69, 1.75, 8.5) (-69, 1.75, -8.5) (-51, 1.75, -8.5) (-51, 1.75, 8.5) (-46, 1.75, 8.5) (-28, 1.75, 8.5) (-28, 1.75, -8.5) (-46, 1.75, -8.5)
fillet "Fillet15" radius 1 4 edges at (-24.5, 1.75, -27.5) (-24.5, 1.75, -12.5) (-24.5, 1.75, 12.5) (-24.5, 1.75, 27.5)
fillet "Fillet16" radius 5 4 edges at (-41.8852, 1.75, -86) (-41.8852, 1.75, -37) (-41.8852, 1.75, 37) (-41.8852, 1.75, 86)
fillet "Fillet17" radius 2 8 edges at (-36.8852, 1.75, -86) (-36.8852, 1.75, -37) (-26.1148, 1.75, -37) (-26.1148, 1.75, -86) (-36.8852, 1.75, 37) (-26.1148, 1.75, 37) (-36.8852, 1.75, 86) (-26.1148, 1.75, 86)
fillet "Fillet18" radius 2 8 edges at (-21.1148, 1.75, -86) (-17, 1.75, -86) (-17, 1.75, -37) (-21.1148, 1.75, -37) (-21.1148, 1.75, 37) (-17, 1.75, 37) (-17, 1.75, 86) (-21.1148, 1.75, 86)
fillet "Fillet19" radius 5 16 edges at (-12, 1.75, -86) (14.0482, 1.75, -86) (14.0482, 1.75, -37) (-12, 1.75, -37) (19, 1.75, -86) (42.9385, 1.75, -86) (42.9385, 1.75, -37) (19, 1.75, -37) (19, 1.75, 37) (19, 1.75, 86) (42.9385, 1.75, 86) (42.9385, 1.75, 37) (-12, 1.75, 37) (-12, 1.75, 86) (14, 1.75, 86) (14, 1.75, 37)
fillet "Fillet20" radius 5 10 edges at (47.9385, 1.75, -86) (58.4, 1.75, -86) (58.4, 1.75, -69) (81, 1.75, -55) (47.9385, 1.75, -37) (47.9385, 1.75, 37) (81, 1.75, 55) (58, 1.75, 69) (47.9385, 1.75, 86) (58, 1.75, 86)
fillet "Fillet21" radius 15 12 edges at (74, 1.75, -37) (81, 1.75, -44) (74, 1.75, -17) (81, 1.75, -10) (81, 1.75, 10) (74, 1.75, 17) (74, 1.75, 37) (81, 1.75, 44) (-11, 1.75, -17) (-18, 1.75, -10) (-18, 1.75, 10) (-11, 1.75, 17)
fillet "Fillet22" radius 1 2 edges at (-47, 1.75, -27.5) (-47, 1.75, 27.5)
body "Solid1"
